counterweight_v1 (Autodesk Fusion 360 design; units mm, degrees)
Autodesk Fusion 360 part; units mm, degrees
sketch "Sketch1" plane through (0, 0, 0) normal (0, 0, 1) x (1, 0, 0) in component "Component"
  circle A0 centre (0, 0) radius 1
  circle A1 centre (0, 0) radius 2.5
  line L0 (0, 0) -> (10, 0) construction
  line L1 (0, 0) -> (-5, 8.6603) construction
  line L2 (0, 0) -> (7.8295, 0) construction
  arc A2 (10, 0) -> (-5, 8.6603) centre (0, 0) ccw
  line L3 (-5, 8.6603) -> (-1.25, 2.1651)
  line L4 (2.5, 0) -> (10, 0)
  line L5 (-1.25, 2.1651) -> (-2.75, 4.7631) construction
  arc A3 (-2.3654, 0.8093) -> (-2.75, 4.7631) centre (-6.9069, 2.3631) ccw
  line L6 (2.5, 0) -> (5.5, 0)
  arc A4 (5.5, 0) -> (1.8836, -1.6438) centre (5.5, -4.8) ccw
  dimension "d1" = 2
  dimension "d2" = 5
  dimension "d3" = 10
  dimension "d4" = 120
  dimension "d5" = 10
  dimension "d6" = 3
  dimension "d7" = 3
  constraint coincident A0.centre A1.centre
  constraint concentric A0 A1
  constraint horizontal L0
  constraint horizontal L2
  constraint coincident A1 L3.end
  constraint coincident L1 L3.end
  constraint coincident L2 L4.start
  constraint coincident A1 L4.start
  constraint parallel L3 L5
  constraint tangent A1 A3
  constraint coincident A1 A3.start
  constraint tangent L5 A3
  constraint parallel L0 L6
  constraint tangent A1 A4
  constraint coincident A1 A4.end
  constraint tangent L0 A4
  measures "d1" diameter of A0
  measures "d2" diameter of A1
  measures "d3" distance of A0.centre L0.end
  measures "d4" angle of L1 L2
  measures "d5" distance of A0.centre L1.end
  measures "d6" distance of L3.end L5.end
  measures "d7" distance of L4.start L6.end
extrude "Extrude1" add sketch "Sketch1" along normal blind 6 in component "Component"
component "Component" placed x (1, 0, 0) y (0, 1, 0) z (0, 0, 1) at (0, 0, 0)
equation "d5 = d3"
